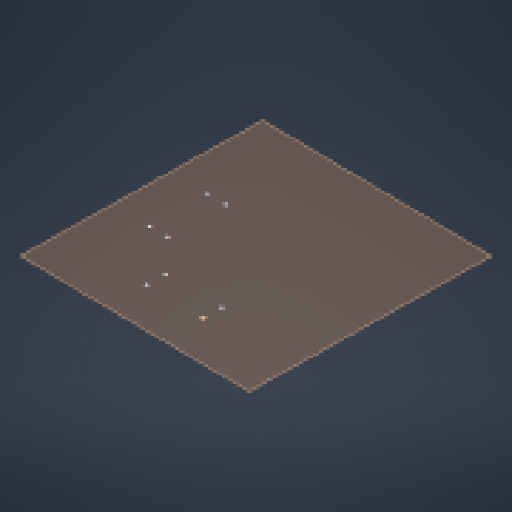
# Autodesk Inventor part: Mesa
Saved by Autodesk Inventor 2024 (Build 280153000, 153)
## iProperties
Created: 2023-04-23
Part Number: Mesa
Material: Genérico
Document SubType Name: Modeling
Designer: javie
Density: 1 g/cm^3
Appearance: Valor por defecto
Author: javie
Autodesk Inventor part; units mm, degrees
ref_plane "YZ Plane" through (0, 0, 0) normal (1, 0, 0) x (0, 1, 0)
ref_plane "XZ Plane" through (0, 0, 0) normal (0, 1, 0) x (-1, 0, 0)
ref_plane "XY Plane" through (0, 0, 0) normal (0, 0, 1) x (1, 0, 0)
ref_plane "Plano de trabajo1" through (5045.3695, -1674.7645, 1275.4449) normal (-0.0021155, 0.9999955, -0.0021345) x (-0.9998916, -0.0021464, -0.0145673)
sketch "Boceto1" plane through (5045.3695, -1674.7645, 1275.4449) normal (-0.0021155, 0.9999955, -0.0021345) x (-0.9998916, -0.0021464, -0.0145673)
  line L0 (-860.5005, 1150.6528) -> (-860.5005, 1750.6528)
  line L1 (-860.5005, 1750.6528) -> (839.4995, 1750.6528)
  line L2 (-13.7894, 1495.6811) -> (-13.7894, 1723.4426)
  line L3 (-780.5005, 1750.6528) -> (-780.5005, 1670.6528)
  circle A0 centre (-795.5005, 1685.6528) radius 5
  circle A1 centre (-795.5005, 1735.6528) radius 5
  circle A2 centre (-845.5005, 1685.6528) radius 5
  circle A3 centre (-845.5005, 1735.6528) radius 5
  line L4 (-780.5005, 1670.6528) -> (-860.5005, 1670.6528)
  line L5 (1423.1842, 863.9864) -> (1423.1842, -832.9469)
  line L6 (823.1842, 863.9864) -> (1423.1842, 863.9864)
  line L7 (1423.1842, 863.9864) -> (1423.1842, 783.9864)
  line L8 (1423.1842, 783.9864) -> (1343.1842, 783.9864)
  line L9 (1343.1842, 783.9864) -> (1343.1842, 863.9864)
  line L10 (1343.1842, 863.9864) -> (1423.1842, 863.9864)
  circle A4 centre (1408.1842, 848.9864) radius 5
  circle A5 centre (1408.1842, 798.9864) radius 5
  circle A6 centre (1358.1842, 848.9864) radius 5
  circle A7 centre (1358.1842, 798.9864) radius 5
  line L11 (-805.5005, 1695.6528) -> (-835.5005, 1695.6528)
  line L12 (-835.5005, 1695.6528) -> (-835.5005, 1725.6528)
  line L13 (-835.5005, 1725.6528) -> (-805.5005, 1725.6528)
  line L14 (-805.5005, 1725.6528) -> (-805.5005, 1695.6528)
  line L15 (1398.1842, 808.9864) -> (1368.1842, 808.9864)
  line L16 (1368.1842, 808.9864) -> (1368.1842, 838.9864)
  line L17 (1368.1842, 838.9864) -> (1398.1842, 838.9864)
  line L18 (1398.1842, 838.9864) -> (1398.1842, 808.9864)
  point P0 (5059.8075, -1198.2636)
  point P1 (1343.1842, 863.9864)
  point P2 (1423.1842, 783.9864)
  point P3 (-820.5005, 1670.6528)
  point P4 (-805.5005, 1710.6528)
  point P5 (1383.1842, 808.9864)
  dimension "d0" = 1700
  dimension "d1" = 600
  dimension "d17" = 80
  dimension "d18" = 80
  dimension "d21" = 10
  dimension "d22" = 15
  dimension "d23" = 15
  dimension "d35" = 30
  dimension "d36" = 30
  dimension "d37" = 25
  dimension "d38" = 25
  dimension "d39" = 30
  dimension "d40" = 30
  dimension "d41" = 25
  dimension "d42" = 25
  dimension "d45" = 15
  dimension "d46" = 15
  dimension "d47" = 15
  dimension "d48" = 15
  dimension "d49" = 15
  dimension "d50" = 15
  dimension "d51" = 15
  constraints: 38 end point, 8 centre point, 6 parallel, 3 midpoint, 3 perpendicular, 2 horizontal, 1 vertical
  measures "d0" distance of L0.end L1.end
  measures "d1" distance of L0.start L0.end
  measures "d17" distance of L8.end L9.end
  measures "d18" distance of L7.end L8.end
  measures "d21" diameter of A4
  measures "d22" distance from line of L5 A4.centre
  measures "d23" distance from line of L6 A4.centre
  measures "d35" distance of L12.end L13.end
  measures "d36" distance of L11.end L12.end
  measures "d37" distance from line of point (-820.501, 1670.653) L11
  measures "d38" distance from line of L3 point (-805.501, 1710.653)
  measures "d39" distance of L16.end L17.end
  measures "d40" distance of L15.end L16.end
  measures "d41" distance from line of L8 point (1383.184, 808.986)
  measures "d42" distance between parallel lines of L9 L16
  measures "d45" distance from line of L9 A6.centre
  measures "d46" distance from line of L10 A6.centre
  measures "d47" distance from line of L10 A4.centre
  measures "d48" distance from line of L5 A5.centre
  measures "d49" distance from line of L8 A5.centre
  measures "d50" distance from line of L8 A7.centre
  measures "d51" distance from line of L9 A7.centre
extrude "Extrusión1" add sketch "Boceto1" along normal blind 6 contours L0 L1 L3 L4 | L5 L8 L9 L6 | L11 L12 L13 L14 | L15 L16 L17 L18
ref_plane "Plano de trabajo2" through (5045.3568, -1668.7646, 1275.4321) normal (-0.0021155, 0.9999955, -0.0021345) x (0.9998916, 0.0021464, 0.0145673)
sketch "Boceto3" plane through (5045.3568, -1668.7646, 1275.4321) normal (-0.0021155, 0.9999955, -0.0021345) x (0.9998916, 0.0021464, 0.0145673)
  line L0 (805.5005, -1695.6528) -> (835.5005, -1695.6528)
  line L1 (835.5005, -1695.6528) -> (835.5005, -1725.6528)
  line L2 (835.5005, -1725.6528) -> (805.5005, -1725.6528)
  line L3 (805.5005, -1725.6528) -> (805.5005, -1695.6528)
  line L4 (860.5005, -1670.6528) -> (780.5005, -1670.6528) projected
  line L5 (780.5005, -1670.6528) -> (780.5005, -1750.6528) projected
  line L6 (-1398.1842, -808.9864) -> (-1368.1842, -808.9864)
  line L7 (-1368.1842, -808.9864) -> (-1368.1842, -838.9864)
  line L8 (-1368.1842, -838.9864) -> (-1398.1842, -838.9864)
  line L9 (-1398.1842, -838.9864) -> (-1398.1842, -808.9864)
  line L10 (-1343.1842, -863.9864) -> (-1343.1842, -783.9864) projected
  line L11 (-1343.1842, -783.9864) -> (-1423.1842, -783.9864) projected
  point P0 (-5059.8075, 1198.2636)
  point P1 (820.5005, -1670.6528)
  point P2 (820.5005, -1695.6528)
  point P3 (780.5005, -1710.6528)
  point P4 (-1343.1842, -823.9864)
  point P5 (-1368.1842, -823.9864)
  point P6 (-1383.1842, -808.9864)
  dimension "d52" = 30
  dimension "d53" = 30
  dimension "d54" = 25
  dimension "d55" = 25
  dimension "d56" = 30
  dimension "d57" = 30
  dimension "d59" = 25
  dimension "d60" = 25
  constraints: 16 end point, 6 midpoint, 4 parallel, 2 horizontal, 2 perpendicular
  measures "d52" distance of L1.end L2.end
  measures "d53" distance of L0.end L1.end
  measures "d54" distance of point (820.501, -1670.653) point (820.501, -1695.653)
  measures "d55" distance from line of point (780.501, -1710.653) L3
  measures "d56" distance of L7.end L8.end
  measures "d57" distance of L6.end L7.end
  measures "d59" distance between parallel lines of L10 L7
  measures "d60" distance from line of L11 point (-1383.184, -808.986)
extrude "Extrusión3" cut sketch "Boceto3" against normal blind 2.5
